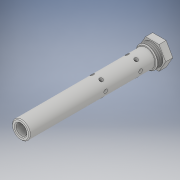
# Autodesk Inventor part: axe_reservoir_bloqueur
Saved by Autodesk Inventor 2019 (Build 230136000, 136)
## iProperties
Created: 2019-03-19
Part Number: axe_reservoir_bloqueur
Material: Générique
Document SubType Name: Modeling
Designer: theor
Density: 1 g/cm^3
Appearance: Par défaut
Author: theor
Autodesk Inventor part; units mm, degrees
ref_plane "YZ Plane" through (0, 0, 0) normal (1, 0, 0) x (0, 1, 0)
ref_plane "XZ Plane" through (0, 0, 0) normal (0, 1, 0) x (-1, 0, 0)
ref_plane "XY Plane" through (0, 0, 0) normal (0, 0, 1) x (1, 0, 0)
sketch "Esquisse1" plane through (0, 0, 0) normal (1, 0, 0) x (0, 1, 0)
  line L0 (0, 0) -> (0, 10.7004)
  line L1 (5, 0) -> (5, -70)
  line L2 (5, -70) -> (6, -70)
  line L3 (6, -70) -> (6, -73.5)
  line L4 (6, -73.5) -> (8, -73.5)
  line L5 (8, -73.5) -> (8, -77.5)
  line L6 (8, -77.5) -> (3, -77.5)
  line L7 (3, -77.5) -> (3, -59)
  line L8 (3, -59) -> (0, -59)
  line L9 (0, -59) -> (0, -55)
  line L10 (0, -55) -> (3, -55)
  line L11 (3, -55) -> (3, 0)
  line L12 (5, 0) -> (3, 0)
  dimension "d0" = 12
  dimension "d1" = 3.5
  dimension "d2" = 4
  dimension "d3" = 2
  dimension "d4" = 6
  dimension "d5" = 10
  dimension "d6" = 11
  dimension "d7" = 4
  dimension "d8" = 2
  dimension "d46" = 70
  constraints: 26 end point, 6 vertical, 5 horizontal, 2 collinear, 2 perpendicular, 1 horizontal alignment
  measures "d0" diameter of L3 L0
  measures "d1" distance of L2.end L3.end
  measures "d2" distance of L4.end L5.end
  measures "d3" distance of L3.end L4.end
  measures "d4" diameter of L7 L0
  measures "d5" diameter of L1 L0
  measures "d6" distance between parallel lines of L2 L8
  measures "d7" distance of L8.end L9.end
  measures "d8" distance between parallel lines of L7 L1
  measures "d46" distance between parallel lines of L12 L2
revolve "Révolution1" add sketch "Esquisse1" angle 360 about axis through (0, 0, 0) along (0, 0, 1)
thread "Filetage1" size "M12x1" class "6g" standard "ISO Metric profile" full length
thread "Filetage2" size "M6x1" class "6H" standard "ISO Metric profile" length 10
sketch "Esquisse2" plane through (0, 0, -77.5) normal (0, 0, -1) x (-1, 0, 0)
  line L0 (3.7528, 6.5) -> (7.5056, 0)
  line L1 (7.5056, 0) -> (3.7528, -6.5)
  line L2 (3.7528, -6.5) -> (-3.7528, -6.5)
  line L3 (-3.7528, -6.5) -> (-7.5056, 0)
  line L4 (-7.5056, 0) -> (-3.7528, 6.5)
  line L5 (-3.7528, 6.5) -> (3.7528, 6.5)
  circle A0 centre (0, 0) radius 3 projected
  circle A1 centre (0, 0) radius 8 projected
  dimension "d15" = 13
  constraints: 12 end point, 1 coincident, 1 horizontal, 13 other
  measures "d15" distance between parallel lines of L2 L5
extrude "Extrusion1" cut sketch "Esquisse2" against normal up to surface (4 mm away) contours A1
chamfer "Chanfrein2" distance 0.5 angle 45 1 edges at (0, -6, -70)
sketch "Esquisse3" plane through (0, 0, 0) normal (1, 0, 0) x (0, 1, 0)
  circle A0 centre (0, -42.5) radius 1
  line L0 (-3, -55) -> (3, -55) projected
  point P0 (0, 0)
  dimension "d24" = 2
  dimension "d42" = 12.5
  constraints: 1 centre point, 1 vertical alignment
  measures "d24" diameter of A0
  measures "d42" distance from line of L0 A0.centre
extrude "Extrusion2" cut sketch "Esquisse3" along normal mid plane 12
sketch "Esquisse5" plane through (0, 0, 0) normal (1, 0, 0) x (0, 1, 0)
  circle A0 centre (0, -62) radius 1
  line L0 (-3, -59) -> (3, -59) projected
  point P0 (0, 0)
  dimension "d38" = 3
  dimension "d39" = 2
  constraints: 1 centre point, 1 vertical alignment
  measures "d38" distance from line of A0.centre L0
  measures "d39" diameter of A0
extrude "Extrusion4" cut sketch "Esquisse5" along normal mid plane 12
pattern_circular "Réseau circulaire1" count 3 over 360 about axis through (0, 0, -10) along (0, 0, 1) of "Extrusion2", "Extrusion4"
chamfer "Chanfrein3" distance 0.5 angle 45 2 edges at (0, -5, 0) (0, -3, 0)
